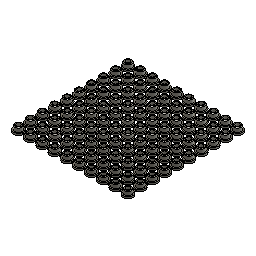
TinyNES_Shoulder_Washer (Autodesk Fusion 360 design; units mm, degrees)
Autodesk Fusion 360 part; units mm, degrees
cylinder "CylinderPrimitive1" add diameter 6.5 height 1.2 placed x (1, 0, 0) y (0, 0, -1) z (0, 1, 0) at (0, 0, 0) makes body 1
hole "Hole1" at (0, 1.2, 0) direction (0, -1, 0) diameter 2.75 end through all bodies 1
sketch "Sketch2" plane through (0, 1.2, 0) normal (0, 1, 0) x (-1, 0, 0)
  circle A0 centre (0, 0) radius 1.375
  circle A1 centre (0, 0) radius 3.25
  circle A2 centre (0, 0) radius 2.375
  dimension "d6" = 4.75
  constraint coincident A0.centre A1.centre
  measures "d6" diameter of A2
extrude "Extrude1" add sketch "Sketch2" along normal blind 2.75 contours A2 bodies 1
chamfer "Chamfer1" distance 0.4 angle 45 1 edges at (2.2143, 3.95, -0.8588) on bodies 1
pattern_linear "R-Pattern1" count 10 spacing 8 along (0, 0, 1) count 10 spacing 8 along (1, 0, 0) of bodies 1 makes body 2 at (-2.372, 2.7667, 7.8816) makes body 3 at (-2.372, 2.7667, 15.8816) makes body 4 at (-2.372, 2.7667, 23.8816) makes body 5 at (-2.372, 2.7667, 31.8816) makes body 6 at (-2.372, 2.7667, 39.8816) makes body 7 at (-2.372, 2.7667, 47.8816) makes body 8 at (-2.372, 2.7667, 55.8816) makes body 9 at (-2.372, 2.7667, 63.8816) makes body 10 at (2.0266, 2.7667, 70.7616) makes body 11 at (5.628, 2.7667, -0.1184) makes body 12 at (5.628, 2.7667, 7.8816) makes body 13 at (5.628, 2.7667, 15.8816) makes body 14 at (5.628, 2.7667, 23.8816) makes body 15 at (5.628, 2.7667, 31.8816) makes body 16 at (5.628, 2.7667, 39.8816) makes body 17 at (5.628, 2.7667, 47.8816) makes body 18 at (5.628, 2.7667, 55.8816) makes body 19 at (5.628, 2.7667, 63.8816) makes body 20 at (10.0266, 2.7667, 70.7616) makes body 21 at (13.628, 2.7667, -0.1184) makes body 22 at (13.628, 2.7667, 7.8816) makes body 23 at (13.628, 2.7667, 15.8816) makes body 24 at (13.628, 2.7667, 23.8816) makes body 25 at (13.628, 2.7667, 31.8816) makes body 26 at (13.628, 2.7667, 39.8816) makes body 27 at (13.628, 2.7667, 47.8816) makes body 28 at (13.628, 2.7667, 55.8816) makes body 29 at (13.628, 2.7667, 63.8816) makes body 30 at (18.0266, 2.7667, 70.7616) makes body 31 at (21.628, 2.7667, -0.1184) makes body 32 at (21.628, 2.7667, 7.8816) makes body 33 at (21.628, 2.7667, 15.8816) makes body 34 at (21.628, 2.7667, 23.8816) makes body 35 at (21.628, 2.7667, 31.8816) makes body 36 at (21.628, 2.7667, 39.8816) makes body 37 at (21.628, 2.7667, 47.8816) makes body 38 at (21.628, 2.7667, 55.8816) makes body 39 at (21.628, 2.7667, 63.8816) makes body 40 at (26.0266, 2.7667, 70.7616) makes body 41 at (29.628, 2.7667, -0.1184) makes body 42 at (29.628, 2.7667, 7.8816) makes body 43 at (29.628, 2.7667, 15.8816) makes body 44 at (29.628, 2.7667, 23.8816) makes body 45 at (29.628, 2.7667, 31.8816) makes body 46 at (29.628, 2.7667, 39.8816) makes body 47 at (29.628, 2.7667, 47.8816) makes body 48 at (29.628, 2.7667, 55.8816) makes body 49 at (29.628, 2.7667, 63.8816) makes body 50 at (34.0266, 2.7667, 70.7616) makes body 51 at (37.628, 2.7667, -0.1184) makes body 52 at (37.628, 2.7667, 7.8816) makes body 53 at (37.628, 2.7667, 15.8816) makes body 54 at (37.628, 2.7667, 23.8816) makes body 55 at (37.628, 2.7667, 31.8816) makes body 56 at (37.628, 2.7667, 39.8816) makes body 57 at (37.628, 2.7667, 47.8816) makes body 58 at (37.628, 2.7667, 55.8816) makes body 59 at (37.628, 2.7667, 63.8816) makes body 60 at (42.0266, 2.7667, 70.7616) makes body 61 at (45.628, 2.7667, -0.1184) makes body 62 at (45.628, 2.7667, 7.8816) makes body 63 at (45.628, 2.7667, 15.8816) makes body 64 at (45.628, 2.7667, 23.8816) makes body 65 at (45.628, 2.7667, 31.8816) makes body 66 at (45.628, 2.7667, 39.8816) makes body 67 at (45.628, 2.7667, 47.8816) makes body 68 at (45.628, 2.7667, 55.8816) makes body 69 at (45.628, 2.7667, 63.8816) makes body 70 at (50.0266, 2.7667, 70.7616) makes body 71 at (53.628, 2.7667, -0.1184) makes body 72 at (53.628, 2.7667, 7.8816) makes body 73 at (53.628, 2.7667, 15.8816) makes body 74 at (53.628, 2.7667, 23.8816) makes body 75 at (53.628, 2.7667, 31.8816) makes body 76 at (53.628, 2.7667, 39.8816) makes body 77 at (53.628, 2.7667, 47.8816) makes body 78 at (53.628, 2.7667, 55.8816) makes body 79 at (53.628, 2.7667, 63.8816) makes body 80 at (58.0266, 2.7667, 70.7616) makes body 81 at (64.7564, 2.7667, 2.2513) makes body 82 at (64.7564, 2.7667, 10.2513) makes body 83 at (64.7564, 2.7667, 18.2513) makes body 84 at (64.7564, 2.7667, 26.2513) makes body 85 at (64.7564, 1.9833, 29.7487) makes body 86 at (64.7564, 2.7667, 42.2513) makes body 87 at (64.7564, 2.7667, 50.2513) makes body 88 at (64.7564, 2.7667, 58.2513) makes body 89 at (64.7564, 2.7667, 66.2513) makes body 90 at (64.7564, 2.7667, 74.2513) makes body 91 at (71.7047, 2.7667, 2.3566) makes body 92 at (71.7047, 1.9833, 5.6434) makes body 93 at (71.7047, 2.7667, 18.3566) makes body 94 at (71.7047, 2.7667, 26.3566) makes body 95 at (71.7047, 2.7667, 34.3566) makes body 96 at (71.7047, 2.7667, 42.3566) makes body 97 at (71.7047, 2.7667, 50.3566) makes body 98 at (71.7047, 2.7667, 58.3566) makes body 99 at (71.7047, 1.9833, 61.6434) makes body 100 at (71.7047, 2.7667, 74.3566)
sketch "Sketch4" plane through (0, 0, 0) normal (0, -1, 0) x (1, 0, 0)
  circle A0 centre (0, 0) radius 1.375
  circle A1 centre (0, 0) radius 3.25
  line L0 (0, 0) -> (0, 8) construction
  line L1 (0.5, 5) -> (-0.5, 5)
  line L2 (-0.5, 5) -> (-0.5, 3)
  line L3 (-0.5, 3) -> (0.5, 3)
  line L4 (0.5, 3) -> (0.5, 5)
  line L5 (0.5, 5) -> (-0.5, 3) construction
  line L6 (-0.5, 5) -> (0.5, 3) construction
  line L7 (0, 0) -> (8, 0) construction
  line L8 (5, 0.5) -> (3, 0.5)
  line L9 (3, 0.5) -> (3, -0.5)
  line L10 (3, -0.5) -> (5, -0.5)
  line L11 (5, -0.5) -> (5, 0.5)
  line L12 (5, 0.5) -> (3, -0.5) construction
  line L13 (3, 0.5) -> (5, -0.5) construction
  point P0 (0, 4)
  point P1 (4, 0)
  dimension "d14" = 8
  dimension "d15" = 1
  dimension "d16" = 2
  dimension "d23" = 8
  dimension "d24" = 2
  dimension "d25" = 1
  constraint coincident A0.centre A1.centre
  constraint vertical L0
  constraint horizontal L1
  constraint perpendicular L1 L2
  constraint parallel L1 L3
  constraint parallel L2 L4
  constraint coincident L5 P0
  constraint coincident L6 P0
  constraint midpoint L0 P0
  constraint perpendicular L0 L7
  constraint horizontal L8
  constraint perpendicular L8 L9
  constraint parallel L8 L10
  constraint parallel L9 L11
  constraint coincident L12 P1
  constraint coincident L13 P1
  constraint midpoint L7 P1
  measures "d14" distance of A0.centre L0.end
  measures "d15" distance of L2.end L3.end
  measures "d16" distance of L1.end L2.end
  measures "d23" distance of A0.centre L7.end
  measures "d24" distance of L9.end L10.end
  measures "d25" distance of L8.end L9.end
extrude "Extrude2" add sketch "Sketch4" against normal blind 0.5 separate body contours A1 L8 L10 L11 | A1 L1 L2 L4 makes body 101 at (0.0558, 0, 4.4152) makes body 102 at (4.4152, 0.5, -0.0558)
pattern_linear "R-Pattern2" count 10 spacing 8 along (1, 0, 0) count 9 spacing 8 along (0, 0, 1) of bodies 101 makes body 103 at (8.0558, 0, 4.4152) makes body 104 at (16.0558, 0, 4.4152) makes body 105 at (24.0558, 0, 4.4152) makes body 106 at (32.0558, 0, 4.4152) makes body 107 at (40.0558, 0, 4.4152) makes body 108 at (48.0558, 0, 4.4152) makes body 109 at (56.0558, 0, 4.4152) makes body 110 at (64.0558, 0, 4.4152) makes body 111 at (72.0558, 0, 4.4152) makes body 112 at (0.0558, 0, 12.4152) makes body 113 at (8.0558, 0, 12.4152) makes body 114 at (16.0558, 0, 12.4152) makes body 115 at (24.0558, 0, 12.4152) makes body 116 at (32.0558, 0, 12.4152) makes body 117 at (40.0558, 0, 12.4152) makes body 118 at (48.0558, 0, 12.4152) makes body 119 at (56.0558, 0, 12.4152) makes body 120 at (64.0558, 0, 12.4152) makes body 121 at (72.0558, 0, 12.4152) makes body 122 at (0.0558, 0, 20.4152) makes body 123 at (8.0558, 0, 20.4152) makes body 124 at (16.0558, 0, 20.4152) makes body 125 at (24.0558, 0, 20.4152) makes body 126 at (32.0558, 0, 20.4152) makes body 127 at (40.0558, 0, 20.4152) makes body 128 at (48.0558, 0, 20.4152) makes body 129 at (56.0558, 0, 20.4152) makes body 130 at (64.0558, 0, 20.4152) makes body 131 at (72.0558, 0, 20.4152) makes body 132 at (0.0558, 0, 28.4152) makes body 133 at (8.0558, 0, 28.4152) makes body 134 at (16.0558, 0, 28.4152) makes body 135 at (24.0558, 0, 28.4152) makes body 136 at (32.0558, 0, 28.4152) makes body 137 at (40.0558, 0, 28.4152) makes body 138 at (48.0558, 0, 28.4152) makes body 139 at (56.0558, 0, 28.4152) makes body 140 at (64.0558, 0, 28.4152) makes body 141 at (72.0558, 0, 28.4152) makes body 142 at (0.0558, 0, 36.4152) makes body 143 at (8.0558, 0, 36.4152) makes body 144 at (16.0558, 0, 36.4152) makes body 145 at (24.0558, 0, 36.4152) makes body 146 at (32.0558, 0, 36.4152) makes body 147 at (40.0558, 0, 36.4152) makes body 148 at (48.0558, 0, 36.4152) makes body 149 at (56.0558, 0, 36.4152) makes body 150 at (64.0558, 0, 36.4152) makes body 151 at (72.0558, 0, 36.4152) makes body 152 at (0.0558, 0, 44.4152) makes body 153 at (8.0558, 0, 44.4152) makes body 154 at (16.0558, 0, 44.4152) makes body 155 at (24.0558, 0, 44.4152) makes body 156 at (32.0558, 0, 44.4152) makes body 157 at (40.0558, 0, 44.4152) makes body 158 at (48.0558, 0, 44.4152) makes body 159 at (56.0558, 0, 44.4152) makes body 160 at (64.0558, 0, 44.4152) makes body 161 at (72.0558, 0, 44.4152) makes body 162 at (0.0558, 0, 52.4152) makes body 163 at (8.0558, 0, 52.4152) makes body 164 at (16.0558, 0, 52.4152) makes body 165 at (24.0558, 0, 52.4152) makes body 166 at (32.0558, 0, 52.4152) makes body 167 at (40.0558, 0, 52.4152) makes body 168 at (48.0558, 0, 52.4152) makes body 169 at (56.0558, 0, 52.4152) makes body 170 at (64.0558, 0, 52.4152) makes body 171 at (72.0558, 0, 52.4152) makes body 172 at (0.0558, 0, 60.4152) makes body 173 at (8.0558, 0, 60.4152) makes body 174 at (16.0558, 0, 60.4152) makes body 175 at (24.0558, 0, 60.4152) makes body 176 at (32.0558, 0, 60.4152) makes body 177 at (40.0558, 0, 60.4152) makes body 178 at (48.0558, 0, 60.4152) makes body 179 at (56.0558, 0, 60.4152) makes body 180 at (64.0558, 0, 60.4152) makes body 181 at (72.0558, 0, 60.4152) makes body 182 at (0.0558, 0, 68.4152) makes body 183 at (8.0558, 0, 68.4152) makes body 184 at (16.0558, 0, 68.4152) makes body 185 at (24.0558, 0, 68.4152) makes body 186 at (32.0558, 0, 68.4152) makes body 187 at (40.0558, 0, 68.4152) makes body 188 at (48.0558, 0, 68.4152) makes body 189 at (56.0558, 0, 68.4152) makes body 190 at (64.0558, 0, 68.4152) makes body 191 at (72.0558, 0, 68.4152)
pattern_linear "R-Pattern3" count 9 spacing 8 along (1, 0, 0) count 10 spacing 8 along (0, 0, 1) of bodies 102 makes body 192 at (12.4152, 0.5, -0.0558) makes body 193 at (20.4152, 0.5, -0.0558) makes body 194 at (28.4152, 0.5, -0.0558) makes body 195 at (36.4152, 0, 0.0558) makes body 196 at (44.4152, 0, 0.0558) makes body 197 at (52.4152, 0, 0.0558) makes body 198 at (60.4152, 0, 0.0558) makes body 199 at (68.4152, 0, 0.0558) makes body 200 at (4.4152, 0.5, 7.9442) makes body 201 at (12.4152, 0.5, 7.9442) makes body 202 at (20.4152, 0.5, 7.9442) makes body 203 at (28.4152, 0.5, 7.9442) makes body 204 at (36.4152, 0, 8.0558) makes body 205 at (44.4152, 0, 8.0558) makes body 206 at (52.4152, 0, 8.0558) makes body 207 at (60.4152, 0, 8.0558) makes body 208 at (68.4152, 0, 8.0558) makes body 209 at (4.4152, 0.5, 15.9442) makes body 210 at (12.4152, 0.5, 15.9442) makes body 211 at (20.4152, 0.5, 15.9442) makes body 212 at (28.4152, 0.5, 15.9442) makes body 213 at (36.4152, 0, 16.0558) makes body 214 at (44.4152, 0, 16.0558) makes body 215 at (52.4152, 0, 16.0558) makes body 216 at (60.4152, 0, 16.0558) makes body 217 at (68.4152, 0, 16.0558) makes body 218 at (4.4152, 0.5, 23.9442) makes body 219 at (12.4152, 0.5, 23.9442) makes body 220 at (20.4152, 0.5, 23.9442) makes body 221 at (28.4152, 0.5, 23.9442) makes body 222 at (36.4152, 0.5, 23.9442) makes body 223 at (44.4152, 0.5, 23.9442) makes body 224 at (52.4152, 0.5, 23.9442) makes body 225 at (60.4152, 0.5, 23.9442) makes body 226 at (68.4152, 0.5, 23.9442) makes body 227 at (4.4152, 0, 32.0558) makes body 228 at (12.4152, 0, 31.9442) makes body 229 at (20.4152, 0, 31.9442) makes body 230 at (28.4152, 0, 31.9442) makes body 231 at (36.4152, 0, 32.0558) makes body 232 at (44.4152, 0, 32.0558) makes body 233 at (52.4152, 0, 32.0558) makes body 234 at (60.4152, 0, 32.0558) makes body 235 at (68.4152, 0, 32.0558) makes body 236 at (4.4152, 0, 40.0558) makes body 237 at (12.4152, 0, 39.9442) makes body 238 at (20.4152, 0, 39.9442) makes body 239 at (28.4152, 0, 39.9442) makes body 240 at (36.4152, 0, 40.0558) makes body 241 at (44.4152, 0, 40.0558) makes body 242 at (52.4152, 0, 40.0558) makes body 243 at (60.4152, 0, 40.0558) makes body 244 at (68.4152, 0, 40.0558) makes body 245 at (4.4152, 0, 48.0558) makes body 246 at (12.4152, 0, 47.9442) makes body 247 at (20.4152, 0, 47.9442) makes body 248 at (28.4152, 0, 47.9442) makes body 249 at (36.4152, 0, 48.0558) makes body 250 at (44.4152, 0, 48.0558) makes body 251 at (52.4152, 0, 48.0558) makes body 252 at (60.4152, 0, 48.0558) makes body 253 at (68.4152, 0, 48.0558) makes body 254 at (4.4152, 0, 56.0558) makes body 255 at (12.4152, 0, 55.9442) makes body 256 at (20.4152, 0, 55.9442) makes body 257 at (28.4152, 0, 55.9442) makes body 258 at (36.4152, 0, 56.0558) makes body 259 at (44.4152, 0, 56.0558) makes body 260 at (52.4152, 0, 56.0558) makes body 261 at (60.4152, 0, 56.0558) makes body 262 at (68.4152, 0, 56.0558) makes body 263 at (4.4152, 0.5, 63.9442) makes body 264 at (12.4152, 0.5, 63.9442) makes body 265 at (20.4152, 0.5, 63.9442) makes body 266 at (28.4152, 0.5, 63.9442) makes body 267 at (36.4152, 0.5, 63.9442) makes body 268 at (44.4152, 0.5, 63.9442) makes body 269 at (52.4152, 0.5, 63.9442) makes body 270 at (60.4152, 0.5, 63.9442) makes body 271 at (68.4152, 0.5, 63.9442) makes body 272 at (4.4152, 0, 71.9442) makes body 273 at (12.4152, 0, 71.9442) makes body 274 at (20.4152, 0, 71.9442) makes body 275 at (28.4152, 0, 71.9442) makes body 276 at (36.4152, 0, 72.0558) makes body 277 at (44.4152, 0, 72.0558) makes body 278 at (52.4152, 0, 72.0558) makes body 279 at (60.4152, 0, 72.0558) makes body 280 at (68.4152, 0, 72.0558)
combine "Combine1" operation add target body 1 tool bodies 23 46 244 51 227 50 271 3 114 27 265 180 122 245 85 109 238 266 179 210 40 219 242 96 86 95 243 233 84 88 83 82 81 251 249 252 130 254 208 258 250 71 80 113 259 76 69 261 255 67 226 74 264 256 257 65 70 68 62 268 59 64 57 274 79 49 41 60 278 37 73 29 52 21 20 17 13 276 19 236 194 61 195 58 135 38 221 34 31 277 108 35 103 102 269 220 164 197 44 144 270 263 262 216 116 124 134 8 168 25 160 203 91 36 273 92 6 156 140 205 218 272 42 185 97 145 170 212 118 153 126 106 211 235 224 26 12 14 133 75 215 101 93 198 166 98 48 78 66 115 4 181 209 63 77 169 162 2 246 11 230 155 72 267 43 24 28 196 279 248 260 143 121 171 136 142 47 32 123 90 184 99 157 30 7 39 9 253 16 56 182 241 117 173 223 188 55 138 127 191 54 137 165 232 53 148 147 192 240 204 222 213 193 5 231 174 152 178 199 177 139 206 172 128 186 129 167 119 187 111 158 112 151 217 150 141 107 131 94 207 105 120 104 214 110 89 159 234 100 87 225 10 18 22 175 132 154 247 163 15 202 149 33 146 228 45 237 229 239 200 183 280 161 190 189 176 275 125 201
